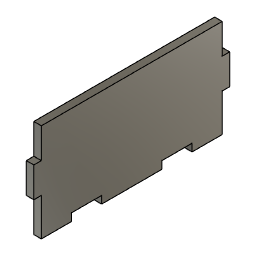
Drawer Back (1x) (Autodesk Fusion 360 design; units mm, degrees)
Autodesk Fusion 360 part; units mm, degrees
sketch "Sketch1" plane through (0, 0, 0) normal (1, 0, 0) x (0, 1, 0)
  line L0 (0, 0) -> (76.2, 0)
  line L1 (0, 0) -> (12.7, 0)
  line L2 (12.7, 0) -> (12.7, -3.175)
  line L3 (12.7, -3.175) -> (0, -3.175)
  line L4 (0, -3.175) -> (0, 0)
  line L5 (12.7, 0) -> (25.4, 0)
  line L6 (25.4, 0) -> (25.4, -3.175)
  line L7 (25.4, -3.175) -> (38.1, -3.175)
  line L8 (76.2, 0) -> (76.2, -3.175)
  line L9 (76.2, -3.175) -> (63.5, -3.175)
  line L10 (63.5, -3.175) -> (63.5, 0)
  line L11 (63.5, 0) -> (50.8, 0)
  line L12 (50.8, 0) -> (50.8, -3.175)
  line L13 (50.8, -3.175) -> (38.1, -3.175)
  line L14 (0, 0) -> (0, 38.1)
  line L15 (0, 38.1) -> (76.2, 38.1)
  line L16 (76.2, 38.1) -> (76.2, 0)
  line L17 (0, 0) -> (0, 12.7)
  line L18 (0, 12.7) -> (-3.175, 12.7)
  line L19 (-3.175, 12.7) -> (-3.175, 25.4)
  line L20 (-3.175, 25.4) -> (0, 25.4)
  line L21 (76.2, 0) -> (76.2, 12.7)
  line L22 (76.2, 12.7) -> (79.375, 12.7)
  line L23 (79.375, 12.7) -> (79.375, 25.4)
  line L24 (79.375, 25.4) -> (76.2, 25.4)
  dimension "d1" = 76.2
  dimension "d2" = 12.7
  dimension "d3" = 3.175
  dimension "d4" = 12.7
  dimension "d5" = 3.175
  dimension "d6" = 12.7
  dimension "d7" = 3.175
  dimension "d8" = 12.7
  dimension "d9" = 12.7
  dimension "d10" = 3.175
  dimension "d11" = 38.1
  dimension "d12" = 12.7
  dimension "d13" = 3.175
  dimension "d14" = 12.7
  dimension "d15" = 12.7
  dimension "d16" = 3.175
  dimension "d17" = 12.7
  constraint coincident L0.start L1.start
  constraint horizontal L0
  constraint parallel L0 L1
  constraint perpendicular L0 L2
  constraint perpendicular L2 L3
  constraint perpendicular L1 L4
  constraint perpendicular L2 L5
  constraint perpendicular L5 L6
  constraint perpendicular L6 L7
  constraint perpendicular L0 L8
  constraint perpendicular L8 L9
  constraint coincident L0 L10.end
  constraint perpendicular L0 L10
  constraint perpendicular L10 L11
  constraint perpendicular L0 L12
  constraint perpendicular L1 L14
  constraint perpendicular L14 L15
  constraint perpendicular L1 L17
  constraint perpendicular L14 L18
  constraint perpendicular L18 L19
  constraint coincident L14 L20.end
  constraint perpendicular L14 L20
  constraint perpendicular L0 L21
  constraint perpendicular L16 L22
  constraint perpendicular L22 L23
  constraint coincident L16 L24.end
  constraint perpendicular L16 L24
  measures "d1" distance of L0.start L0.end
  measures "d2" distance of L0.start L1.end
  measures "d3" distance of L1.end L2.end
  measures "d4" distance of L1.end L5.end
  measures "d5" distance of L5.end L6.end
  measures "d6" distance of L6.end L7.end
  measures "d7" distance of L0.end L8.end
  measures "d8" distance of L8.end L9.end
  measures "d9" distance of L10.end L11.end
  measures "d10" distance of L11.end L12.end
  measures "d11" distance of L0.start L14.end
  measures "d12" distance of L0.start L17.end
  measures "d13" distance of L17.end L18.end
  measures "d14" distance of L18.end L19.end
  measures "d15" distance of L0.end L21.end
  measures "d16" distance of L21.end L22.end
  measures "d17" distance of L22.end L23.end
extrude "Extrude1" add sketch "Sketch1" along normal blind 3.175
